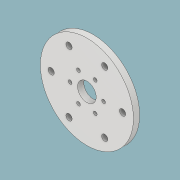
# Autodesk Inventor part: TA04
Saved by Autodesk Inventor 2017 SP1 (Build 210196100, 196)
## iProperties
Created: 2018-10-09
Part Number: TA04
Material: ABS Plastic
Document SubType Name: Modeling
Designer: Zach
Density: 1.06 g/cm^3
Appearance: Smooth - White
Author: Zach
Autodesk Inventor part; units mm, degrees
ref_plane "YZ Plane" through (0, 0, 0) normal (1, 0, 0) x (0, 1, 0)
ref_plane "XZ Plane" through (0, 0, 0) normal (0, 1, 0) x (-1, 0, 0)
ref_plane "XY Plane" through (0, 0, 0) normal (0, 0, 1) x (1, 0, 0)
sketch "Sketch1" plane through (0, 0, 0) normal (0, 0, 1) x (1, 0, 0)
  circle A0 centre (0, 0) radius 37.5
  circle A1 centre (0, 0) radius 7.5
  circle A2 centre (28.75, 0) radius 2.5
  circle A3 centre (13.5, 0) radius 1.5
  circle A4 centre (14.375, 24.8982) radius 2.5
  circle A5 centre (6.75, 11.6913) radius 1.5
  circle A6 centre (-14.375, 24.8982) radius 2.5
  circle A7 centre (-6.75, 11.6913) radius 1.5
  circle A8 centre (-28.75, 0) radius 2.5
  circle A9 centre (-13.5, 0) radius 1.5
  circle A10 centre (-14.375, -24.8982) radius 2.5
  circle A11 centre (-6.75, -11.6913) radius 1.5
  circle A12 centre (14.375, -24.8982) radius 2.5
  circle A13 centre (6.75, -11.6913) radius 1.5
  dimension "d0" = 75
  dimension "d1" = 15
  dimension "d2" = 5
  dimension "d3" = 3
  dimension "d4" = 28.75
  dimension "d5" = 13.5
  dimension "d8" = 360
  constraints: 14 centre point, 2 coincident, 2 horizontal alignment, 25 other
  measures "d0" diameter of A0
  measures "d1" diameter of A1
  measures "d2" diameter of A2
  measures "d3" diameter of A3
  measures "d4" distance of point (0, 0) A2.centre
  measures "d5" distance of point (0, 0) A3.centre
extrude "Extrusion1" add sketch "Sketch1" along normal blind 5
body "Solid1"
